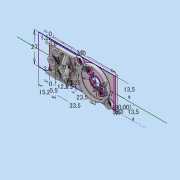
# Autodesk Inventor part: B3board
Saved by Autodesk Inventor 2022 (Build 260153000, 153)
## iProperties
Created: 2024-04-23
Part Number: B3board
Material: 一般
Document SubType Name: Modeling
Designer: ktamu
Density: 1 g/cm^3
Appearance: 既定
Author: ktamu
Autodesk Inventor part; units mm, degrees
ref_plane "YZ Plane" through (0, 0, 0) normal (1, 0, 0) x (0, 1, 0)
ref_plane "XZ Plane" through (0, 0, 0) normal (0, 1, 0) x (-1, 0, 0)
ref_plane "XY Plane" through (0, 0, 0) normal (0, 0, 1) x (1, 0, 0)
sketch "BASEscetch" plane through (0, 0, 0) normal (0, 0, 1) x (1, 0, 0)
  line L0 (-30, 13.6) -> (30, -13.6) construction
  line L1 (30, 13.6) -> (-30, -13.6) construction
  circle A0 centre (21.0963, 0) radius 4.35
  circle A1 centre (21.0963, 0) radius 13.5
  circle A2 centre (21.0963, 0) radius 12.24
  line L2 (39.5823, -8) -> (39.5823, -6.0137) construction
  line L3 (39.5963, -13.5) -> (39.5963, 13.5)
  line L4 (39.5963, 13.5) -> (-20.4037, 13.5)
  line L5 (-20.4037, 13.5) -> (-20.4037, -13.5)
  line L6 (-20.4037, -13.5) -> (39.5963, -13.5)
  line L7 (39.5963, -13.5) -> (66.5963, -13.5) construction
  circle A3 centre (-2.4037, 0) radius 2
  circle A4 centre (-14.9037, 0) radius 2
  line L8 (-49.4437, 0) -> (85.9363, 0) projected
  circle A5 centre (-11.1677, -8.9) radius 2
  line L9 (-1.6537, 12.5) -> (-3.1537, 12.5)
  line L10 (-3.1537, -12.5) -> (-1.6537, -12.5)
  line L11 (-1.6537, 12.5) -> (-3.1537, -12.5) construction
  line L12 (-3.1537, 12.5) -> (-1.6537, -12.5) construction
  line L13 (0.1463, -12.5) -> (-20.4037, -12.5)
  circle A6 centre (-11.1677, -8.9) radius 3.5
  circle A7 centre (-11.1677, 8.9) radius 2
  circle A8 centre (-11.1677, 8.9) radius 3.5
  circle A9 centre (-14.9037, 0) radius 3.5
  circle A10 centre (-2.4037, 0) radius 3.5
  circle A11 centre (7.78, 10) radius 3.5
  circle A12 centre (7.78, 10) radius 2.8
  line L14 (21.0963, 0) -> (28.731, -7.6346) construction
  line L15 (21.0963, 0) -> (31.8933, 0) construction
  line L16 (-30.1037, 13.5) -> (-30.1037, -13.5)
  line L17 (-30.1037, 13.5) -> (-20.4037, 13.5)
  line L18 (-30.1037, -13.5) -> (-20.4037, -13.5)
  circle A13 centre (7.78, 10) radius 1.5
  line L19 (-20.4037, -12.5) -> (-20.4037, -13.5)
  line L20 (5.3305, 12.5) -> (-20.4037, 12.5)
  line L21 (-3.1537, 11) -> (-3.1537, 3.4187)
  line L22 (-1.6537, 3.4187) -> (-1.6537, 11)
  line L23 (-1.6537, -11) -> (-1.6537, -3.4187)
  line L24 (-3.1537, -3.4187) -> (-3.1537, -11)
  circle A14 centre (34.6012, -10) radius 3.5
  circle A15 centre (34.6012, -10) radius 2.8
  circle A16 centre (34.6012, -10) radius 1.5
  line L25 (21.0963, 0) -> (39.5893, -18.493) construction
  line L26 (38.1012, -13.5) -> (38.1012, 13.5)
  line L27 (0.1463, -12.5) -> (0.1463, -11)
  line L28 (0.1463, -11) -> (-20.4177, -11)
  line L29 (-20.4177, -11) -> (-20.4177, -12.5)
  line L30 (-20.4177, -12.5) -> (0.1463, -12.5)
  line L31 (3.3963, -11) -> (3.3963, -13.5) construction
  line L32 (4.4259, 11) -> (-20.4037, 11)
  line L33 (13.5359, 7.0446) -> (14.2686, 7.7251)
  line L34 (17.0951, 7.6208) -> (17.5576, 7.1228)
  line L35 (17.4532, 4.2963) -> (16.7205, 3.6158)
  line L36 (13.894, 3.7202) -> (13.4315, 4.2181)
  line L37 (11.9703, 5.4231) -> (12.9703, 5.4231) construction
  arc A17 (13.5359, 7.0446) -> (13.4315, 4.2181) centre (14.897, 5.5792) ccw
  arc A18 (17.0951, 7.6208) -> (14.2686, 7.7251) centre (15.6297, 6.2597) ccw
  arc A19 (17.4532, 4.2963) -> (17.5576, 7.1228) centre (16.0922, 5.7618) ccw
  arc A20 (13.894, 3.7202) -> (16.7205, 3.6158) centre (15.3595, 5.0812) ccw
  circle A21 centre (21.0963, 0) radius 5.25
  line L38 (25.0236, -4.4541) -> (25.7563, -3.7736)
  line L39 (28.5828, -3.8779) -> (29.0453, -4.3759)
  line L40 (28.941, -7.2024) -> (28.2083, -7.8829)
  line L41 (25.3817, -7.7786) -> (24.9193, -7.2806)
  line L42 (23.458, -6.0756) -> (24.458, -6.0756) construction
  arc A22 (25.0236, -4.4541) -> (24.9193, -7.2806) centre (26.3847, -5.9195) ccw
  arc A23 (28.5828, -3.8779) -> (25.7563, -3.7736) centre (27.1174, -5.239) ccw
  arc A24 (28.941, -7.2024) -> (29.0453, -4.3759) centre (27.5799, -5.7369) ccw
  arc A25 (25.3817, -7.7786) -> (28.2083, -7.8829) centre (26.8472, -6.4175) ccw
  point P0 (0, 0)
  point P1 (31.8249, -7.8687)
  point P2 (-13.9677, 11)
  point P3 (-8.3677, 11)
  point P4 (-8.3677, -11)
  point P5 (-13.9677, -11)
  point P6 (-20.4037, -11)
  point P7 (9.5364, 6.9726)
  point P8 (11.1771, 9.1574)
  point P9 (31.2986, -8.841)
  point P10 (32.5291, -7.1792)
  point P11 (15.6064, 8.8551)
  point P12 (19.8775, 6.2556)
  point P13 (27.0941, -2.6436)
  dimension "d42" = 7
  dimension "d2" = 8.7
  dimension "d3" = 27
  dimension "d4" = 24.48
  dimension "d11" = 90
  dimension "d12" = 60
  dimension "d13" = 4
  dimension "d14" = 4
  dimension "d16" = 12.5
  dimension "d17" = 0
  dimension "d18" = 23.5
  dimension "d19" = 4
  dimension "d20" = 1.5
  dimension "d22" = 1
  dimension "d23" = 0
  dimension "d24" = 0
  dimension "d25" = 7
  dimension "d27" = 0
  dimension "d28" = 13.5
  dimension "d29" = 13.5
  dimension "d30" = 7
  dimension "d31" = 7
  dimension "d32" = 7
  dimension "d33" = 5.6
  dimension "d34" = 3.5
  dimension "d35" = 45
  dimension "d36" = 27
  dimension "d37" = 15.2
  dimension "d38" = 3
  dimension "d40" = 5.5
  dimension "d41" = 0
  dimension "d43" = 5.6
  dimension "d44" = 3
  dimension "d45" = 3.5
  dimension "d50" = 1.5
  dimension "d51" = 33.5
  dimension "d52" = 3.25
  dimension "d53" = 1.5
  dimension "d54" = 3.6
  dimension "d55" = 3.6
  dimension "d78" = 5
  dimension "d80" = 5
  dimension "d81" = 2
  dimension "d82" = 10.5
  dimension "d83" = 5
  dimension "d84" = 2
  constraints: 84 end point, 25 centre point, 22 point on circle, 16 tangent, 15 parallel, 14 coincident, 12 point on line, 11 perpendicular, 6 equal radius, 5 horizontal, 4 equal length, 4 midpoint, 2 symmetric about line, 2 vertical, 5 other
  measures "d2" diameter of A0
  measures "d3" diameter of A1
  measures "d4" diameter of A2
  measures "d11" angle of L7 L3
  measures "d12" distance of L4.end L3.end
  measures "d13" diameter of A3
  measures "d14" diameter of A4
  measures "d16" distance of A3.centre A4.centre
  measures "d17" distance from line of A0.centre L8
  measures "d18" distance of A3.centre A0.centre
  measures "d19" diameter of A5
  measures "d20" distance of L10.end L10.start
  measures "d22" distance from line of L6 L13.start
  measures "d23" distance from line of L13.end L5
  measures "d24" distance between parallel lines of L13 L10
  measures "d25" diameter of A6
  measures "d27" distance from line of L8 A3.centre
  measures "d28" distance between parallel lines of L6 L8
  measures "d29" distance between parallel lines of L8 L4
  measures "d30" diameter of A9
  measures "d31" diameter of A10
  measures "d32" diameter of A11
  measures "d33" diameter of A12
  measures "d34" distance from line of L4 A11.centre
  measures "d35" angle of L14 L15
  measures "d36" distance of L16.start L16.end
  measures "d37" distance from line of L16 A4.centre
  measures "d38" diameter of A13
  measures "d40" distance from line of A9.centre L5
  measures "d41" distance from line of L5 L20.end
  measures "d43" diameter of A15
  measures "d44" diameter of A16
  measures "d45" distance from line of L6 point (34.601, -10)
  measures "d50" distance of L13.start L27.end
  measures "d51" distance between parallel lines of L31 L16
  measures "d52" distance between parallel lines of L31 L27
  measures "d53" distance between parallel lines of L32 L20
  measures "d54" distance from line of L20 A8.centre
  measures "d55" distance from line of L13 A6.centre
  measures "d78" distance of L37.start point (15.606, 8.855)
  measures "d80" distance of point (15.606, 8.855) point (19.878, 6.256)
  measures "d81" radius of A17
  measures "d82" diameter of A21
  measures "d83" distance of L42.start point (27.094, -2.644)
  measures "d84" radius of A22
extrude "押し出し1" add sketch "BASEscetch" along normal blind 7 contours A10 L8 A3 | L8 A3 A10
extrude "押し出し2" add sketch "BASEscetch" along normal blind 3.5 contours L32 A8 | A8 L32 | L28 A6 | A6 L28 | A9 L8 A4 | L8 A4 A9
extrude "押し出し3mm" add sketch "BASEscetch" along normal blind 3 contours L8 A1 A14 A2 | A2 L8 A1 A11 | A1 A14 | A1 A11 | L32 A8 L5 L20 L9 A11 | L5 L28 A6 L27 L13 L10 picked at (31.9174, -7.8697) picked at (10.3979, 8.0341)
extrude "押し出し4" add sketch "BASEscetch" along normal blind 2 contours A14 A1 | A1 A14 | A11 A1 picked at (10.7523, 8.9847)
extrude "押し出し5" add sketch "BASEscetch" along normal blind 1 contours A12 | A15
extrude "押し出し6" add sketch "BASEscetch" along normal blind 6.5 contours A10 L21 L32 L22
chamfer "面取り1" distance 5.5 distance2 3 1 edges at (-2.4037, 11, 6.5) measured on face at (-2.4037, 10.5, 6.5)
mirror "ミラー1" about plane through (0, 0, 0) normal (0, 1, 0) of "押し出し6"
chamfer "面取り2" distance 3 distance2 5.5 1 edges at (-2.4037, -11, 6.5) measured on face at (-2.4037, -11, 6)
extrude "押し出し7" add sketch "BASEscetch" against normal blind 3.5 contours A10 L8 A3 | L8 A3 A10 | L32 A8 | A8 L32 | L28 A6 | A6 L28 | A9 L8 A4 | L8 A4 A9
extrude "押し出し8" cut sketch "BASEscetch" along normal blind 1 contours A12
extrude "押し出し9" add sketch "BASEscetch" against normal blind 1 contours A12
extrude "押し出し10" add sketch "BASEscetch" against normal blind 2 contours L8 A21 A0 | A0 L8 A21 | A21 L8 A2 | L8 A2 A21 | L8 A1 A14 A2 | A2 L8 A1 A11 | L8 L26 A14 A1 | A1 L4 L26 L8 | L8 A10 L22 L32 A11 A1 | A1 L6 L5 L13 L10 L27 L28 L23 A10 L8 | A1 A11 L4 | A14 A1 | A1 A14 | L26 L4 L3 L8 | L8 L3 L6 L26 | A11 A1 | A1 A11 | A1 A14 L6 | A11 L20 L9 L5 L4 | L26 L6 A14 | L32 A8 L5 L20 L9 A11 | A10 L21 L32 L22 | L23 L28 L24 A10 | L5 L28 A6 L27 L13 L10 | A10 L8 A9 L5 L32 A8 L21 | L24 L28 A6 L5 L8 A9 A10 | A15 | L33 A18 L34 A19 L35 A20 L36 A17 | L38 A23 L39 A24 L40 A25 L41 A22
extrude "押し出し11" cut sketch "BASEscetch" against normal through all contours L33 A18 L34 A19 L35 A20 L36 A17 | L38 A23 L39 A24 L40 A25 L41 A22
chamfer "面取り3" distance 0.9 angle 45 1 edges at (16.7463, 0, 0)
